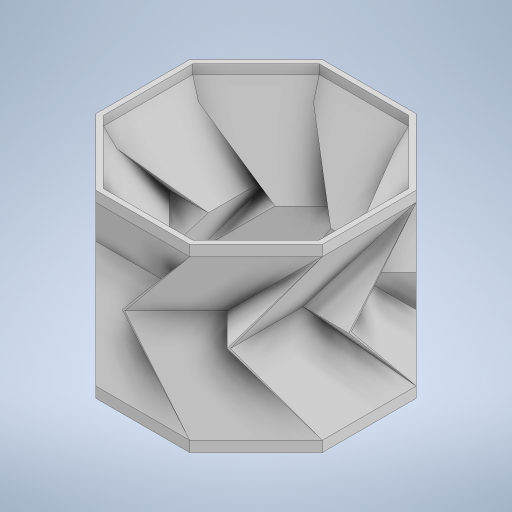
# Autodesk Inventor part: 팔각형 OV-PAM 층 한개
Saved by Autodesk Inventor 2024 (Build 280153000, 153)
## iProperties
Created: 2023-06-16
Part Number: 팔각형 OV-PAM 층 한개
Material: 일반
Document SubType Name: Modeling
Designer: jsw
Density: 1 g/cm^3
Appearance: 기본값
Author: jsw
Autodesk Inventor part; units mm, degrees
ref_plane "YZ Plane" through (0, 0, 0) normal (1, 0, 0) x (0, 1, 0)
ref_plane "XZ Plane" through (0, 0, 0) normal (0, 1, 0) x (-1, 0, 0)
ref_plane "XY Plane" through (0, 0, 0) normal (0, 0, 1) x (1, 0, 0)
sketch "스케치1" plane through (0, 0, 0) normal (0, 1, 0) x (-1, 0, 0)
  line L0 (-12.222, 5.0625) -> (-5.0625, 12.222)
  line L1 (-5.0625, 12.222) -> (5.0625, 12.222)
  line L2 (5.0625, 12.222) -> (12.222, 5.0625)
  line L3 (12.222, 5.0625) -> (12.222, -5.0625)
  line L4 (12.222, -5.0625) -> (5.0625, -12.222)
  line L5 (5.0625, -12.222) -> (-5.0625, -12.222)
  line L6 (-5.0625, -12.222) -> (-12.222, -5.0625)
  line L7 (-12.222, -5.0625) -> (-12.222, 5.0625)
  line L8 (-5.311, 12.822) -> (5.311, 12.822)
  line L9 (5.311, 12.822) -> (12.822, 5.311)
  line L10 (12.822, 5.311) -> (12.822, -5.311)
  line L11 (12.822, -5.311) -> (5.311, -12.822)
  line L12 (5.311, -12.822) -> (-5.311, -12.822)
  line L13 (-5.311, -12.822) -> (-12.822, -5.311)
  line L14 (-12.822, -5.311) -> (-12.822, 5.311)
  line L15 (-12.822, 5.311) -> (-5.311, 12.822)
  point P0 (0, 0)
  point P1 (0, 0)
  point P2 (0, 0)
  dimension "d0" = 10.125
  dimension "d2" = 0.6
  constraints: 32 end point, 2 coincident, 2 horizontal, 34 other
  measures "d0" distance of L0.end L1.end
  measures "d2" distance between parallel lines of L10 L3
extrude "돌출2" add sketch "스케치1" along normal blind 9 contours L0 L1 L2 L3 L4 L5 L6 L7 | L8 L9 L10 L11 L12 L13 L14 L15
ref_plane "작업 평면2" through (12.822, 0, 5.311) normal (-0.8660254, -0.5, 0) x (0, 0, -1)
sketch "스케치3" plane through (12.822, 0, 5.311) normal (1, 0, 0) x (0, 0, -1)
  line L0 (0, 0) -> (0, 9) projected
  line L1 (0, 9) -> (10.6221, 9) projected
  line L2 (0, 0) -> (10.6221, 0)
  line L3 (10.6221, 0) -> (10.6221, 9)
  line L4 (10.6221, 9) -> (0, 9)
  line L5 (0, 9) -> (0, 0)
  line L6 (0, 9) -> (-5.4785, 9)
  line L7 (-7.5109, 9) -> (0, 9) projected
  line L8 (0, 0) -> (-5.4785, 9)
  line L9 (10.6221, 9) -> (5.311, 9)
  line L10 (10.6221, 0) -> (3, 9)
  point P0 (5.311, 0)
  point P1 (-1.4, 12)
  dimension "d17" = 121.33
  dimension "d55" = 3
  constraints: 16 end point, 6 midpoint, 2 parallel, 2 point on line, 1 horizontal, 1 perpendicular
  measures "d17" angle of L8 L2
  measures "d55" distance of L0.end L10.end
extrude "돌출4" cut sketch "스케치3" against normal up to surface contours L8 L6 L0 | L0 L1 L10 L2 surface through (12.822, 0, 5.311) normal (-0.8660254, -0.5, 0)
pattern_circular "원형 패턴1" count 8 over 360 about axis through (0, -10, 0) along (0, 1, 0) of "돌출4"
mirror "미러5" about plane through (0, 9, 0) normal (0, 1, 0) of "돌출2", "돌출4", "원형 패턴1"
sketch "스케치9" plane through (-5.311, 18, -12.822) normal (0, 1, 0) x (1, 0, 0)
  line L0 (18.133, -18.133) -> (18.133, -7.5109) projected
  line L1 (18.133, -7.5109) -> (10.6221, 0) projected
  line L2 (10.6221, 0) -> (0, 0) projected
  line L3 (0, 0) -> (-7.5109, -7.5109) projected
  line L4 (-7.5109, -7.5109) -> (-7.5109, -18.133) projected
  line L5 (-7.5109, -18.133) -> (0, -25.6439) projected
  line L6 (0, -25.6439) -> (10.6221, -25.6439) projected
  line L7 (10.6221, -25.6439) -> (18.133, -18.133) projected
  point P0 (5.311, -12.822)
extrude "돌출8" add sketch "스케치9" along normal blind 1.2
sketch "스케치10" plane through (0, 0, 0) normal (0, -1, 0) x (1, 0, 0)
  line L0 (12.822, 5.311) -> (12.822, -5.311) projected
  line L1 (5.311, 12.822) -> (12.822, 5.311) projected
  line L2 (-5.311, 12.822) -> (5.311, 12.822) projected
  line L3 (-12.822, 5.311) -> (-5.311, 12.822) projected
  line L4 (-12.822, -5.311) -> (-12.822, 5.311) projected
  line L5 (-5.311, -12.822) -> (-12.822, -5.311) projected
  line L6 (5.311, -12.822) -> (-5.311, -12.822) projected
  line L7 (12.822, -5.311) -> (5.311, -12.822) projected
  point P0 (0, 0)
extrude "돌출9" add sketch "스케치10" along normal blind 1.2
shell "쉘6" thickness 0.6 removed faces 2 at (1.7703, 19.2, -0.7333) at (1.7703, -1.2, 4.274)
